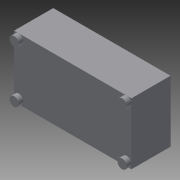
# Autodesk Inventor part: czujnik
Saved by Autodesk Inventor 2014 (Build 180170000, 170)
## iProperties
Created: 2014-12-22
Part Number: czujnik
Material: Ogólny
Document SubType Name: Modeling
Designer: Kuba
Density: 1 g/cm^3
Appearance: Domyślna
Author: Kuba
Autodesk Inventor part; units mm, degrees
ref_plane "YZ Plane" through (0, 0, 0) normal (1, 0, 0) x (0, 1, 0)
ref_plane "XZ Plane" through (0, 0, 0) normal (0, 1, 0) x (-1, 0, 0)
ref_plane "XY Plane" through (0, 0, 0) normal (0, 0, 1) x (1, 0, 0)
sketch "Szkic1" plane through (0, 0, 0) normal (0, 1, 0) x (-1, 0, 0)
  line L0 (63, -33) -> (-63, -33)
  line L1 (-63, -33) -> (-63, 33)
  line L2 (-63, 33) -> (63, 33)
  line L3 (63, 33) -> (63, -33)
  line L4 (63, -33) -> (-63, 33) construction
  line L5 (-63, -33) -> (63, 33) construction
  point P0 (0, 0)
  dimension "d0" = 126
  dimension "d1" = 66
  constraints: 12 end point, 2 midpoint, 2 parallel, 1 horizontal, 1 perpendicular
  measures "d0" distance of L1.end L2.end
  measures "d1" distance of L0.end L1.end
extrude "Wyciągnięcie proste1" add sketch "Szkic1" along normal blind 42
sketch "Szkic2" plane through (0, 0, 0) normal (0, -1, 0) x (1, 0, 0)
  line L0 (-63, -33) -> (63, -33) projected
  line L1 (63, -33) -> (63, 33) projected
  line L2 (63, 33) -> (-63, 33) projected
  line L3 (-63, 33) -> (-63, -33) projected
  line L4 (-58, 28) -> (58, 28)
  line L5 (58, 28) -> (58, -28)
  line L6 (58, -28) -> (-58, -28)
  line L7 (-58, -28) -> (-58, 28)
  circle A0 centre (-58, 28) radius 5
  circle A1 centre (58, 28) radius 5
  circle A2 centre (58, -28) radius 5
  circle A3 centre (-58, -28) radius 5
  point P0 (0, 0)
  dimension "d4" = 5
  dimension "d5" = 10
  dimension "d6" = 10
  dimension "d7" = 10
  dimension "d8" = 10
  constraints: 8 end point, 4 centre point, 4 coincident, 3 other
  measures "d4" distance between parallel lines of L2 L4
  measures "d5" diameter of A0
  measures "d6" diameter of A1
  measures "d7" diameter of A2
  measures "d8" diameter of A3
extrude "Wyciągnięcie proste2" add sketch "Szkic2" along normal blind 5 contours A3 L7 L6 | A2 L6 L5 | L6 L7 A3 | A0 L4 L7 | A2 L5 L6 | L7 L4 A0 | A1 L5 L4 | A1 L4 L5
equation "\"d5\" = 2 * d4"
equation "\"d6\" = 2 * d4"
equation "\"d7\" = 2 * d4"
equation "\"d8\" = 2 * d4"
equation "\"d9\" = d4"
